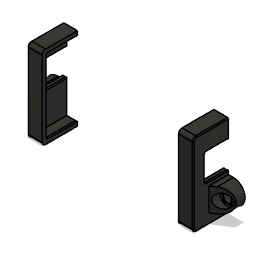
wheel PSU mounts v1 (Autodesk Fusion 360 design; units mm, degrees)
Autodesk Fusion 360 part; units mm, degrees
sketch "Sketch1" plane through (0, 0, 0) normal (1, 0, 0) x (0, 0, -1)
  line L0 (-15.6, 37.4) -> (15.6, 37.4)
  line L1 (15.6, 37.4) -> (15.6, -37.4)
  line L2 (15.6, -37.4) -> (-15.6, -37.4)
  line L3 (-15.6, -37.4) -> (-15.6, 37.4)
  line L4 (-15.6, 37.4) -> (15.6, -37.4) construction
  line L5 (15.6, 37.4) -> (-15.6, -37.4) construction
  line L6 (15.6, 23.4) -> (-8.4, 23.4)
  line L7 (-8.4, 23.4) -> (-8.4, -3.6)
  line L8 (-8.4, -3.6) -> (15.6, -3.6)
  line L9 (15.6, -3.6) -> (15.6, 23.4)
  line L10 (15.6, 37.4) -> (15.6, 42.4)
  line L11 (15.6, 42.4) -> (-20.6, 42.4)
  line L12 (-20.6, 42.4) -> (-20.6, -42.4)
  line L13 (-20.6, -42.4) -> (15.6, -42.4)
  line L14 (15.6, -42.4) -> (15.6, -37.4)
  line L15 (-15.6, -20) -> (15.6, -20) construction
  line L16 (15.6, -8) -> (-4.4, -8)
  line L17 (-4.4, -8) -> (-4.4, -32)
  line L18 (-4.4, -32) -> (15.6, -32)
  line L19 (15.6, -32) -> (15.6, -8)
  dimension "d1" = 74.8
  dimension "d2" = 31.2
  dimension "d3" = 14
  dimension "d4" = 41
  dimension "d5" = 24
  dimension "d6" = 5
  dimension "d7" = 5
  dimension "d8" = 5
  dimension "d9" = 20
  dimension "d10" = 20
  dimension "d11" = 12
  dimension "d12" = 12
  constraint horizontal L0
  constraint perpendicular L0 L1
  constraint parallel L0 L2
  constraint parallel L1 L3
  constraint coincident L4 origin
  constraint coincident L5 origin
  constraint horizontal L6
  constraint vertical L7
  constraint horizontal L8
  constraint vertical L9
  constraint coincident L1 L6.start
  constraint perpendicular L0 L10
  constraint perpendicular L10 L11
  constraint perpendicular L11 L12
  constraint perpendicular L12 L13
  constraint perpendicular L2 L14
  constraint coincident L3 L15.start
  constraint coincident L1 L15.end
  constraint perpendicular L1 L15
  constraint horizontal L16
  constraint vertical L17
  constraint horizontal L18
  constraint vertical L19
  constraint coincident L1 L16.start
  measures "d1" distance of L0.end L1.end
  measures "d2" distance of L0.start L0.end
  measures "d3" distance of L0 L6
  measures "d4" distance of L0 L8
  measures "d5" distance of L6.start L6.end
  measures "d6" distance of L3 L12
  measures "d7" distance of L0 L11
  measures "d8" distance of L2 L13
  measures "d9" distance of origin L15
  measures "d10" distance of L16.start L16.end
  measures "d11" distance of L15 L16
  measures "d12" distance of L15 L18
extrude "Extrude1" add sketch "Sketch1" along normal blind 5 contours L0 L2 L3 L10 L11 L12 L13 L14 | L0 L1 L2 L3 L6 L7 L8 L16 L17 L18 | L1 L16 L17 L18 L19 makes body 1
extrude "Extrude2" add sketch "Sketch1" against normal blind 10 contours L0 L2 L3 L10 L11 L12 L13 L14 bodies 1
extrude "Extrude3" add sketch "Sketch1" along normal blind 22 contours L1 L16 L17 L18 L19 bodies 1
chamfer "Chamfer1" distance 10.8 distance2 17 1 edges at (22, -20, 4.4) measured on face at (22, -24, -8.9333) on bodies 1
sketch "Sketch2" plane through (0, 0, -15.6) normal (0, 0, -1) x (-1, 0, 0)
  line L0 (-5, -32) -> (-5, -42.4)
  line L1 (-5, -42.4) -> (10, -42.4)
  line L2 (10, -42.4) -> (10, -37.4)
  line L3 (10, -37.4) -> (0, -37.4)
  line L4 (0, -37.4) -> (0, -3.6)
  line L5 (0, -3.6) -> (-5, -3.6)
  line L6 (-5, -3.6) -> (-5, -8)
  line L7 (-5, -8) -> (-22, -8)
  line L8 (-22, -8) -> (-22, -32)
  line L9 (-22, -32) -> (-5, -32)
  line L10 (-5, -8) -> (-22, -32) construction
  circle A0 centre (-13.5, -20) radius 4.25
  circle A1 centre (-13.5, -20) radius 7
  dimension "d21" = 8.5
  dimension "d22" = 14
  constraint coincident L6.end L7.start
  constraint coincident L8.end L9.start
  constraint midpoint L10 A0.centre
  constraint concentric A0 A1
  measures "d21" diameter of A0
  measures "d22" diameter of A1
extrude "Extrude4" cut sketch "Sketch2" against normal blind 33 contours A0 | A1 bodies 1
extrude "Extrude5" add sketch "Sketch2" against normal blind 10 contours A1 bodies 1
fillet "Fillet1" radius 12 2 edges at (22, -8, -11) (22, -32, -11) on bodies 1
fillet "Fillet1" radius 1 19 edges at (-5, 37.4, 15.6) (-5, -37.4, 15.6) (-5, 37.4, -15.6) (0, 30.4, -15.6) (0, -20.5, -15.6) (-5, -37.4, -15.6) (-10, -37.4, 0) (-10, 37.4, 0) (-10, 0, 15.6) (2.5, -3.6, 8.4) (2.5, 23.4, 8.4) (0, 23.4, -3.6) (5, 23.4, -3.6) (2.5, 23.4, -15.6) (0, 9.9, 8.4) (5, 9.9, 8.4) (0, -3.6, -3.6) (5, -3.6, -3.6) (2.5, -3.6, -15.6) on bodies 1
fillet "Fillet1" radius 3.5 2 edges at (-2.5, 42.4, 20.6) (-2.5, -42.4, 20.6) on bodies 1
fillet "Fillet1" radius 1 3 edges at (5, 42.4, 2.5) (5, 0, 20.6) (5, -42.4, 2.5) on bodies 1
sketch "Sketch3" plane through (0, 0, -5.6) normal (0, 0, 1) x (1, 0, 0)
  circle A0 centre (13.5, -20) radius 4.25
  circle A1 centre (13.5, -20) radius 7
  line L0 (9.25, -14.4379) -> (9.25, -25.5621)
  line L1 (17.75, -14.4379) -> (17.75, -25.5621)
  line L2 (9.25, -15.75) -> (17.75, -15.75)
  line L3 (9.25, -24.25) -> (17.75, -24.25)
  line L4 (11.7396, -15.75) -> (9.25, -18.2396)
  line L5 (15.2604, -15.75) -> (17.75, -18.2396)
  line L6 (17.75, -21.7604) -> (15.2604, -24.25)
  line L7 (11.7396, -24.25) -> (9.25, -21.7604)
  dimension "d33" = 45
  constraint coincident A1 L0.start
  constraint coincident A1 L0.end
  constraint vertical L0
  constraint coincident A1 L1.start
  constraint coincident A1 L1.end
  constraint parallel L0 L1
  constraint tangent A0 L1
  constraint tangent A0 L0
  constraint coincident L0 L2.start
  constraint coincident L1 L2.end
  constraint perpendicular L1 L2
  constraint coincident L0 L3.start
  constraint coincident L1 L3.end
  constraint perpendicular L1 L3
  constraint tangent A0 L3
  constraint tangent A0 L2
  constraint coincident L2 L4.start
  constraint coincident L0 L4.end
  constraint coincident L2 L5.start
  constraint coincident L1 L5.end
  constraint perpendicular L4 L5
  constraint coincident L1 L6.start
  constraint coincident L3 L6.end
  constraint perpendicular L5 L6
  constraint coincident L3 L7.start
  constraint coincident L0 L7.end
  constraint perpendicular L6 L7
  constraint tangent A0 L4
  constraint tangent A0 L5
  constraint tangent A0 L6
  constraint tangent A0 L7
  measures "d33" angle of L2 L4
extrude "Extrude6" cut sketch "Sketch3" against normal blind 0.2 contours A0 L1 L6 | A0 L1 L5 | A0 L2 L5 | L1 L2 L5 | A0 L3 L6 | L1 L3 L6 | A0 L2 L4 | A1 L0 L1 L2 | A0 L3 L7 | A1 L0 L1 L3 | L0 L2 L4 | A0 L0 L4 | A0 L0 L7 | L0 L3 L7 bodies 1
extrude "Extrude7" cut sketch "Sketch3" against normal blind 0.4 contours A0 L1 L6 | A0 L1 L5 | A0 L2 L5 | L1 L2 L5 | A0 L3 L6 | L1 L3 L6 | A0 L2 L4 | A0 L3 L7 | L0 L2 L4 | A0 L0 L4 | A0 L0 L7 | L0 L3 L7 bodies 1
extrude "Extrude8" cut sketch "Sketch3" against normal blind 0.6 contours A0 L1 L6 | A0 L1 L5 | A0 L2 L5 | A0 L3 L6 | A0 L2 L4 | A0 L3 L7 | A0 L0 L4 | A0 L0 L7 bodies 1
ref_plane "WorkPlane1" through (-80, 0, 0.5) normal (-1, 0, 0) x (0, 0, 1)
mirror "Mirror1" about plane through (-80, 0, 0.5) normal (-1, 0, 0) of bodies 1 makes body 2
copy_body "Body->Comp1" bodies 1 removing the originals makes body 3 in component "wheel PSU mount RH"
copy_body "Body->Comp2" bodies 2 removing the originals makes body 4 in component "wheel PSU mount LH"
component "wheel PSU mount RH" placed x (1, 0, 0) y (0, 1, 0) z (0, 0, 1) at (0, 0, 0)
component "wheel PSU mount LH" placed x (1, 0, 0) y (0, 1, 0) z (0, 0, 1) at (0, 0, 0)
named bodies: "wheel PSU mount RH", "wheel PSU mount LH"
